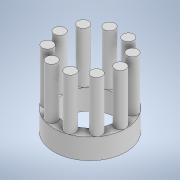
# Autodesk Inventor part: piece_roue_test_2
Saved by Autodesk Inventor 2020.1 (Build 241239000, 239)
## iProperties
Created: 2019-07-25
Part Number: piece_roue_test_2
Material: Générique
Document SubType Name: Modeling
Designer: marlo
Density: 1 g/cm^3
Appearance: Par défaut
Author: marlo
Autodesk Inventor part; units mm, degrees
ref_plane "YZ Plane" through (0, 0, 0) normal (1, 0, 0) x (0, 1, 0)
ref_plane "XZ Plane" through (0, 0, 0) normal (0, 1, 0) x (-1, 0, 0)
ref_plane "XY Plane" through (0, 0, 0) normal (0, 0, 1) x (1, 0, 0)
sketch "Esquisse1" plane through (0, 0, 0) normal (0, 1, 0) x (-1, 0, 0)
  circle A0 centre (0, 0) radius 2.65
  dimension "d0" = 5.3
  constraints: 1 centre point, 1 coincident
  measures "d0" diameter of A0
extrude "Extrusion1" add sketch "Esquisse1" along normal blind 25
sketch "Esquisse2" plane through (0, 0, 0) normal (0, -1, 0) x (1, 0, 0)
  line L0 (2.65, 5.0753) -> (2.65, -12.6206) construction
  circle A0 centre (0, 0) radius 2.65 projected
  circle A1 centre (-14.85, 0) radius 17.5
  line L1 (8.7278, 0) -> (-17.8614, 0) construction
  point P0 (2.65, 0)
  dimension "d4" = 35
  constraints: 4 end point, 2 point on line, 2 tangent, 1 centre point, 1 horizontal, 1 vertical
  measures "d4" diameter of A1
extrude "Extrusion2" add sketch "Esquisse2" along normal blind 10
sketch "Esquisse3" plane through (-14.85, 0, 0) normal (0, 1, 0) x (1, 0, 0)
  line L0 (-17.5, -20.7984) -> (-17.5, 1.736) construction
  circle A0 centre (-12.0139, 8.7286) radius 2.65
  circle A1 centre (-14.85, 0) radius 2.65
  circle A2 centre (-4.5889, 14.1232) radius 2.65
  line L1 (-4.5889, 14.1232) -> (-12.0139, 8.7286) construction
  line L2 (-12.0139, 8.7286) -> (-14.85, 0) construction
  line L3 (-14.85, 0) -> (0, 0) construction
  line L4 (-12.0139, 8.7286) -> (0, 0) construction
  line L5 (-4.5889, 14.1232) -> (0, 0) construction
  line L6 (-14.85, 0) -> (-17.5, 0) construction
  line L7 (-12.0139, 8.7286) -> (-14.1601, 10.283) construction
  line L8 (-4.5889, 14.1232) -> (-6.9476, 15.3312) construction
  line L9 (0, 30.0966) -> (0, -33.1039)
  line L10 (-38.7679, 0) -> (42.4396, 0)
  circle A3 centre (12.0139, 8.7286) radius 2.65
  circle A4 centre (4.5889, 14.1232) radius 2.65
  circle A5 centre (-12.0139, -8.7286) radius 2.65
  circle A6 centre (-4.5889, -14.1232) radius 2.65
  circle A7 centre (4.5889, -14.1232) radius 2.65
  circle A8 centre (12.0139, -8.7286) radius 2.65
  dimension "d14" = 5.3
  constraints: 22 end point, 6 centre point, 6 symmetric about line, 5 equal length, 3 vertical, 2 horizontal, 1 horizontal alignment, 14 other
extrude "Extrusion3" add sketch "Esquisse3" along normal blind 25
sketch "Esquisse4" plane through (-14.85, -10, 0) normal (0, -1, 0) x (1, 0, 0)
  circle A0 centre (14.85, 0) radius 2.65
  constraints: 1 centre point, 1 coincident
extrude "Extrusion4" add sketch "Esquisse4" against normal blind 10
sketch "Esquisse5" plane through (0, 0, 0) normal (0, 1, 0) x (1, 0, 0)
  circle A0 centre (-14.85, 0) radius 12.2
  arc A1 (-9.4422, 16.6435) -> (-20.2578, 16.6435) centre (-14.85, 0) ccw projected
  circle A2 centre (-2.8361, 8.7286) radius 2.65 projected
  point P0 (0, 0)
  constraints: 1 centre point, 1 concentric, 1 tangent
extrude "Extrusion5" cut sketch "Esquisse5" against normal blind 10 contours A0
